nixal_reprap4040_Yidler (Autodesk Fusion 360 design; units mm, degrees)
Autodesk Fusion 360 part; units mm, degrees
sketch "Sketch1" plane through (0, 0, 0) normal (0, 1, 0) x (1, 0, 0)
  line L0 (41, 31) -> (41, -3)
  line L1 (-29, 23) -> (41, 23)
  circle A0 centre (21, -2) radius 1.65
  line L2 (41, 31) -> (-29, 31)
  line L3 (-3.1, 31) -> (-3.1, 35.4)
  line L4 (-3.1, 35.4) -> (5.1, 35.4)
  line L5 (5.1, 35.4) -> (5.1, 31)
  line L6 (5.1, 31) -> (-3.1, 35.4) construction
  line L7 (-3.1, 31) -> (5.1, 35.4) construction
  line L8 (36.5, 13.5) -> (5.5, 13.5) construction
  line L9 (5.5, 13.5) -> (5.5, -17.5) construction
  line L10 (5.5, -17.5) -> (36.5, -17.5) construction
  line L11 (36.5, -17.5) -> (36.5, 13.5) construction
  line L12 (36.5, 13.5) -> (5.5, -17.5) construction
  line L13 (5.5, 13.5) -> (36.5, -17.5) construction
  line L14 (-29, 31) -> (-29, 23)
  line L15 (19.0675, -12) -> (32, -12)
  line L16 (10.0675, -3.0004) -> (10.0664, 23)
  circle A1 centre (21, -2) radius 3.5
  circle A2 centre (21, -2) radius 4
  circle A3 centre (21, -2) radius 6.5
  arc A4 (10.0675, -3.0004) -> (19.0675, -12) centre (19.0675, -3) ccw
  arc A5 (32, -12) -> (41, -3) centre (32, -3) ccw
  dimension "d18" = 20
  dimension "d23" = 3.3
  dimension "d45" = 4.4
  dimension "d46" = 8.2
  dimension "d51" = 31
  dimension "d67" = 41
  dimension "d112" = 70
  dimension "d113" = 40
  dimension "d114" = 2.2
  dimension "d115" = 8
  dimension "d117" = 10
  dimension "d123" = 7
  dimension "d136" = 8
  dimension "d144" = 13
  dimension "d148" = 9
  dimension "d149" = 9
  constraint horizontal L2
  constraint vertical L0
  constraint perpendicular L0 L1
  constraint perpendicular L2 L3
  constraint parallel L2 L4
  constraint parallel L3 L5
  constraint coincident L6 origin
  constraint coincident L7 origin
  constraint parallel L8 L10
  constraint parallel L9 L11
  constraint horizontal L8
  constraint coincident L12 origin
  constraint coincident L13 origin
  constraint vertical L14
  constraint coincident L2
  constraint coincident L0
  constraint coincident L1
  constraint perpendicular L9 L15
  constraint concentric A0 A1
  constraint concentric A1 A2
  constraint concentric A2 A3
  constraint tangent L16 A4
  constraint tangent L15 A4
  constraint tangent L0 A5
  constraint tangent L15 A5
  measures "d18" distance of L0 origin
  measures "d23" diameter of A0
  measures "d67" distance of origin L0
  measures "d112" distance of L0 L14
  measures "d113" distance of L0 origin
  measures "d114" distance of L2 origin
  measures "d115" distance of L1 L2
  measures "d123" diameter of A1
  measures "d136" diameter of A2
  measures "d144" diameter of A3
  measures "d148" radius of A4
  measures "d149" radius of A5
sketch "Sketch2" plane through (0, 0, -23) normal (0, 0, 1) x (1, 0, 0)
  line L0 (41, 8) -> (41, 26)
  line L1 (41, 26) -> (-19, 26)
  circle A0 centre (-14, 17) radius 4
  circle A1 centre (-14, 17) radius 7.5
  line L2 (-19, 26) -> (-19, 8)
  line L3 (-19, 8) -> (41, 8)
  dimension "d31" = 8
  dimension "d32" = 55
  dimension "d33" = 9
  dimension "d36" = 15
  constraint concentric A0 A1
  measures "d31" diameter of A0
  measures "d32" distance of L0 origin
  measures "d33" distance of L1 origin
  measures "d36" diameter of A1
extrude "Extrude12" add sketch "Sketch1" along normal blind 26 and the other way blind 35 contours L0 L1 L2 L14 makes body 1
extrude "Extrude13" cut sketch "Sketch2" against normal blind 28 contours A0 bodies 1
extrude "Extrude14" cut sketch "Sketch2" against normal blind 2 contours A1 L2 | A1 L2 bodies 1
extrude "Extrude15" add sketch "Sketch1" along normal blind 8 contours L0 L1 L15 L16 A4 A5 | A1 | A2 | A3 bodies 1
extrude "Extrude16" add sketch "Sketch1" along normal blind -16 and the other way blind 8 separate body contours L0 L1 L15 L16 A4 A5 | A1 | A2 | A3 makes body 2
extrude "Extrude17" cut sketch "Sketch1" along normal blind 17 and the other way blind -5 contours A1 bodies 1
extrude "Extrude18" cut sketch "Sketch1" along normal blind -32 and the other way blind 12 contours A1 bodies 2
sketch "Sketch4" plane through (0, 0, 0) normal (0, 0, 1) x (1, 0, 0)
  circle A0 centre (-14, -24.9358) radius 4
  circle A1 centre (-14, -24.9358) radius 7.5
  line L0 (41, -35) -> (41, 0)
  dimension "d130" = 8
  dimension "d131" = 15
  dimension "d150" = 55
  constraint concentric A0 A1
  measures "d130" diameter of A0
  measures "d131" diameter of A1
extrude "Extrude19" cut sketch "Sketch4" against normal blind 80 contours A0 bodies 1
extrude "Extrude20" cut sketch "Sketch4" against normal blind 25 bodies 1
extrude "Extrude21" add sketch "Sketch1" against normal blind 1.5 contours A1 | A2 bodies 1
extrude "Extrude22" add sketch "Sketch1" along normal blind -8 and the other way blind 6.5 separate body contours A1 | A2 makes body 3
fillet "Fillet1" radius 2 1 edges at (17.2707, -1.5, 0.5535) on bodies 1
fillet "Fillet2" radius 2 1 edges at (17.2707, -6.5, 0.5535) on bodies 3
extrude "Extrude23" add sketch "Sketch1" along normal blind -6.5 and the other way blind 1.5 separate body contours A1 | A3 makes body 4 at (27.4919, -4.8333, 2.324) makes body 5 at (24.4956, -4.8333, 2.1745)
hidden bodies 4 5
